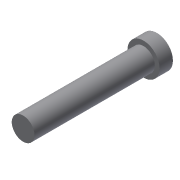
# Autodesk Inventor part: bolt
Saved by Autodesk Inventor 2022 (Build 260148000, 148)
## iProperties
Created: 2006-05-17
Part Number: bolt
Document SubType Name: Modeling
Designer: dchu
Density: 1 g/cm^3
Material: Generic
Appearance: Default
Author: dchu
Autodesk Inventor part; units mm, degrees
ref_plane "YZ Plane" through (0, 0, 0) normal (1, 0, 0) x (0, 1, 0)
ref_plane "XZ Plane" through (0, 0, 0) normal (0, 1, 0) x (-1, 0, 0)
ref_plane "XY Plane" through (0, 0, 0) normal (0, 0, 1) x (1, 0, 0)
sketch "Sketch1" plane through (0, 0, 0) normal (0, 0, 1) x (1, 0, 0)
  line L0 (0, -20.0171) -> (0, 79.9829)
  line L1 (0, 79.9829) -> (12, 79.9829)
  line L2 (12, 79.9829) -> (12, 69.9829)
  line L3 (12, 69.9829) -> (8.5, 69.9829)
  line L4 (8.5, 69.9829) -> (8.5, -20.0171)
  line L5 (8.5, -20.0171) -> (0, -20.0171)
  dimension "d0" = 12
  dimension "d1" = 8.5
  dimension "d4" = 90
  dimension "d6" = 100
  constraints: 12 end point, 4 parallel, 1 perpendicular, 1 vertical
  measures "d0" distance between parallel lines of L0 L2
  measures "d1" distance between parallel lines of L0 L4
  measures "d4" distance of L3.end L4.end
  measures "d6" distance between parallel lines of L5 L1
revolve "Revolution1" add sketch "Sketch1" angle 360 about axis through (0, -20.0171, 0) along (0, 1, 0)
body "Solid1"
